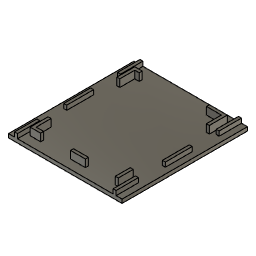
ArduinostandV4 (Autodesk Fusion 360 design; units mm, degrees)
Autodesk Fusion 360 part; units mm, degrees
sketch "Sketch1" plane through (0, 0, 0) normal (0, 0, 1) x (1, 0, 0)
  line L0 (0, 0) -> (76, 0)
  line L1 (76, 0) -> (76, 84)
  line L2 (76, 84) -> (0, 84)
  line L3 (0, 84) -> (0, 0)
  dimension "d1" = 76
  dimension "d2" = 84
  constraint horizontal L0
  constraint vertical L1
  constraint horizontal L2
  constraint vertical L3
  constraint coincident L0.start L3.end
  measures "d1" distance of L0.start L0.end
  measures "d2" distance of L0.start L2.end
extrude "Extrude1" add sketch "Sketch1" along normal blind 2.5
sketch "Sketch2" plane through (0, 0, 2.5) normal (0, 0, 1) x (-1, 0, 0)
  line L0 (0, -84) -> (0, 0)
  line L1 (0, 0) -> (-76, 0)
  line L2 (-76, 0) -> (-76, -84)
  line L3 (-76, -84) -> (0, -84)
  line L4 (0, -84) -> (-4, -84)
  line L5 (-4, -84) -> (-6, -84)
  line L6 (-6, -84) -> (-6, -69)
  line L7 (-6, -69) -> (-4, -69)
  line L8 (-4, -69) -> (-4, -84)
  line L9 (-4, -69) -> (-4, -51)
  line L10 (-4, -51) -> (-6, -51)
  line L11 (-6, -51) -> (-6, -33)
  line L12 (-6, -33) -> (-4, -33)
  line L13 (-4, -33) -> (-4, -51)
  line L14 (-4, -33) -> (-4, -15)
  line L15 (-4, -15) -> (-6, -15)
  line L16 (-6, -15) -> (-6, 0)
  line L17 (-6, 0) -> (-4, 0)
  line L18 (-4, 0) -> (-4, -15)
  line L19 (-6, -84) -> (-40, -84)
  line L20 (-4, -84) -> (-38, -84)
  line L21 (-38, -84) -> (-38, -65)
  line L22 (-72, -69) -> (-72, -84)
  line L23 (-70, -84) -> (-70, -69)
  line L24 (-72, -84) -> (-38, -84)
  line L25 (-70, -69) -> (-72, -69)
  line L26 (-72, -51) -> (-70, -51)
  line L27 (-70, -51) -> (-70, -33)
  line L28 (-72, -33) -> (-72, -51)
  line L29 (-70, -33) -> (-72, -33)
  line L30 (-72, -15) -> (-70, -15)
  line L31 (-70, -15) -> (-70, 0)
  line L32 (-72, 0) -> (-72, -15)
  line L33 (-70, 0) -> (-72, 0)
  dimension "d5" = 4
  dimension "d6" = 2
  dimension "d7" = 15
  dimension "d8" = 18
  dimension "d9" = 2
  dimension "d10" = 18
  dimension "d11" = 18
  dimension "d12" = 2
  dimension "d13" = 15
  dimension "d15" = 34
  constraint coincident L0.start L3.end
  constraint perpendicular L0 L4
  constraint horizontal L5
  constraint vertical L6
  constraint horizontal L7
  constraint vertical L8
  constraint perpendicular L7 L9
  constraint horizontal L10
  constraint vertical L11
  constraint horizontal L12
  constraint vertical L13
  constraint perpendicular L12 L14
  constraint horizontal L15
  constraint vertical L16
  constraint horizontal L17
  constraint vertical L18
  constraint perpendicular L6 L19
  constraint perpendicular L8 L20
  constraint perpendicular L20 L21
  constraint symmetric L4.end L21 L22.end
  constraint symmetric L5.end L21 L23.start
  constraint symmetric L6.end L21 L23.end
  constraint symmetric L7.end L21 L22.start
  constraint symmetric L9.end L21 L26.start
  constraint symmetric L10.end L21 L26.end
  constraint symmetric L11.end L21 L27.end
  constraint symmetric L12.end L21 L28.start
  constraint symmetric L14.end L21 L30.start
  constraint symmetric L15.end L21 L30.end
  constraint symmetric L16.end L21 L31.end
  constraint symmetric L17.end L21 L32.start
  constraint symmetric L20.end L21 L24.end
  measures "d5" distance of L0.start L4.end
  measures "d6" distance of L4.end L5.end
  measures "d7" distance of L4.end L7.end
  measures "d8" distance of L7.end L9.end
  measures "d9" distance of L9.end L10.end
  measures "d10" distance of L9.end L12.end
  measures "d11" distance of L12.end L14.end
  measures "d12" distance of L14.end L15.end
  measures "d13" distance of L14.end L17.end
  measures "d15" distance of L4.end L20.end
extrude "Extrude2" add sketch "Sketch2" along normal blind 3 contours L3 L5 L6 L7 L8 L20 | L1 L15 L16 L17 L18 | L10 L11 L12 L13 | L1 L30 L31 L32 L33 | L3 L22 L23 L24 L25 | L26 L27 L28 L29
sketch "Sketch3" plane through (0, 0, 2.5) normal (0, 0, 1) x (-1, 0, 0)
  line L0 (-72, -15) -> (-72, 0)
  line L1 (-72, 0) -> (-76, 0)
  line L2 (-76, 0) -> (-76, -84)
  line L3 (-76, -84) -> (-72, -84)
  line L4 (-72, -84) -> (-72, -69)
  line L5 (-72, -69) -> (-70, -69)
  line L6 (-70, -69) -> (-70, -84)
  line L7 (-70, -84) -> (-6, -84)
  line L8 (-6, -84) -> (-6, -69)
  line L9 (-6, -69) -> (-4, -69)
  line L10 (-4, -69) -> (-4, -84)
  line L11 (-4, -84) -> (0, -84)
  line L12 (0, -84) -> (0, 0)
  line L13 (0, 0) -> (-4, 0)
  line L14 (-4, 0) -> (-4, -15)
  line L15 (-4, -15) -> (-6, -15)
  line L16 (-6, -15) -> (-6, 0)
  line L17 (-6, 0) -> (-70, 0)
  line L18 (-70, 0) -> (-70, -15)
  line L19 (-70, -15) -> (-72, -15)
  line L20 (-4, -33) -> (-4, -51)
  line L21 (-4, -51) -> (-6, -51)
  line L22 (-6, -51) -> (-6, -33)
  line L23 (-6, -33) -> (-4, -33)
  line L24 (-70, -33) -> (-70, -51)
  line L25 (-70, -51) -> (-72, -51)
  line L26 (-72, -51) -> (-72, -33)
  line L27 (-72, -33) -> (-70, -33)
  line L28 (-70, -84) -> (-67.5, -84)
  line L29 (-67.5, -84) -> (-67.5, -79)
  line L30 (-67.5, -79) -> (-55.5, -79)
  line L31 (-55.5, -79) -> (-55.5, -77)
  line L32 (-55.5, -77) -> (-67.5, -77)
  line L33 (-67.5, -77) -> (-67.5, -79)
  line L34 (-67.5, -77) -> (-65.5, -77)
  line L35 (-65.5, -77) -> (-65.5, -67)
  line L36 (-65.5, -67) -> (-67.5, -67)
  line L37 (-67.5, -67) -> (-67.5, -77)
  line L38 (-67.5, -79) -> (-8.5, -79)
  line L39 (-8.5, -79) -> (-8.5, -76)
  line L40 (-8.5, -76) -> (-13.5, -76)
  line L41 (-13.5, -76) -> (-13.5, -74)
  line L42 (-13.5, -74) -> (-8.5, -74)
  line L43 (-8.5, -74) -> (-8.5, -76)
  line L44 (-8.5, -74) -> (-10.5, -74)
  line L45 (-10.5, -74) -> (-10.5, -64)
  line L46 (-10.5, -64) -> (-8.5, -64)
  line L47 (-8.5, -64) -> (-8.5, -74)
  line L48 (-67.5, -67) -> (-67.5, -16)
  line L49 (-67.5, -16) -> (-65.5, -16)
  line L50 (-65.5, -16) -> (-65.5, -6)
  line L51 (-65.5, -6) -> (-67.5, -6)
  line L52 (-67.5, -6) -> (-67.5, -16)
  line L53 (-65.5, -6) -> (-45.5, -6)
  line L54 (-45.5, -6) -> (-35.5, -6)
  line L55 (-35.5, -6) -> (-35.5, -8)
  line L56 (-35.5, -8) -> (-45.5, -8)
  line L57 (-45.5, -8) -> (-45.5, -6)
  line L58 (-35.5, -6) -> (-15.5, -6)
  line L59 (-15.5, -6) -> (-8.5, -6)
  line L60 (-8.5, -6) -> (-8.5, -8)
  line L61 (-8.5, -8) -> (-15.5, -8)
  line L62 (-15.5, -8) -> (-15.5, -6)
  line L63 (-8.5, -8) -> (-10.5, -8)
  line L64 (-10.5, -8) -> (-10.5, -18)
  line L65 (-10.5, -18) -> (-8.5, -18)
  line L66 (-8.5, -18) -> (-8.5, -8)
  dimension "d19" = 2.5
  dimension "d20" = 5
  dimension "d21" = 12
  dimension "d22" = 2
  dimension "d23" = 2
  dimension "d24" = 10
  dimension "d25" = 59
  dimension "d26" = 3
  dimension "d27" = 5
  dimension "d28" = 2
  dimension "d29" = 10
  dimension "d30" = 51
  dimension "d31" = 2
  dimension "d32" = 10
  dimension "d33" = 20
  dimension "d34" = 10
  dimension "d35" = 2
  dimension "d36" = 20
  dimension "d37" = 7
  dimension "d38" = 2
  dimension "d39" = 2
  dimension "d40" = 10
  constraint coincident L6.end L7.start
  constraint perpendicular L6 L28
  constraint perpendicular L7 L29
  constraint horizontal L30
  constraint vertical L31
  constraint horizontal L32
  constraint vertical L33
  constraint horizontal L34
  constraint vertical L35
  constraint horizontal L36
  constraint vertical L37
  constraint perpendicular L31 L38
  constraint perpendicular L38 L39
  constraint horizontal L40
  constraint vertical L41
  constraint horizontal L42
  constraint vertical L43
  constraint horizontal L44
  constraint vertical L45
  constraint horizontal L46
  constraint vertical L47
  constraint perpendicular L36 L48
  constraint horizontal L49
  constraint vertical L50
  constraint horizontal L51
  constraint vertical L52
  constraint perpendicular L50 L53
  constraint horizontal L54
  constraint vertical L55
  constraint horizontal L56
  constraint vertical L57
  constraint perpendicular L55 L58
  constraint horizontal L59
  constraint vertical L60
  constraint horizontal L61
  constraint vertical L62
  constraint horizontal L63
  constraint vertical L64
  constraint horizontal L65
  constraint vertical L66
  measures "d19" distance of L6.end L28.end
  measures "d20" distance of L28.end L29.end
  measures "d21" distance of L29.end L30.end
  measures "d22" distance of L29.end L32.end
  measures "d23" distance of L32.end L34.end
  measures "d24" distance of L32.end L36.end
  measures "d25" distance of L29.end L38.end
  measures "d26" distance of L38.end L39.end
  measures "d27" distance of L39.end L40.end
  measures "d28" distance of L42.end L44.end
  measures "d29" distance of L42.end L46.end
  measures "d30" distance of L36.end L48.end
  measures "d31" distance of L48.end L49.end
  measures "d32" distance of L48.end L51.end
  measures "d33" distance of L50.end L53.end
  measures "d34" distance of L53.end L54.end
  measures "d35" distance of L53.end L56.end
  measures "d36" distance of L54.end L58.end
  measures "d37" distance of L58.end L59.end
  measures "d38" distance of L58.end L61.end
  measures "d39" distance of L60.end L63.end
  measures "d40" distance of L60.end L65.end
extrude "Extrude3" add sketch "Sketch3" along normal blind 5 contours L30 L31 L32 L33 L34 L38 | L32 L34 L35 L36 L37 | L40 L41 L42 L43 L44 | L42 L44 L45 L46 L47 | L49 L50 L51 L52 | L54 L55 L56 L57 | L59 L60 L61 L62 L63 | L61 L63 L64 L65 L66
